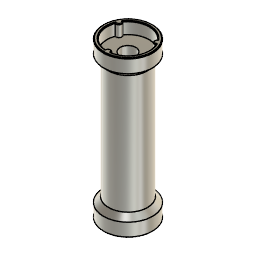
10 Spool Top Hat for Voron 2.4 - Alpha Release (Autodesk Fusion 360 archive; units mm, degrees)
design "spool roller"
Autodesk Fusion 360 part; units mm, degrees
sketch "Sketch1" plane through (0, 0, 0) normal (0, 0, 1) x (1, 0, 0)
  circle A0 centre (0, 0) radius 12.5
  circle A1 centre (0, 0) radius 14.5
  dimension "d1" = 25
  dimension "d2" = 2
  constraint coincident A0.centre A1.centre
  measures "d1" diameter of A0
extrude "Extrude1" add sketch "Sketch1" along normal blind 7
sketch "Sketch2" plane through (0, 0, 0) normal (0, 0, -1) x (1, 0, 0)
  circle A0 centre (0, 0) radius 12.5
  circle A1 centre (0, 0) radius 14.5
extrude "Extrude2" add sketch "Sketch2" along normal blind 1 contours A0 | A1
sketch "Sketch3" plane through (0, 0, -1) normal (0, 0, -1) x (1, 0, 0)
  circle A0 centre (0, 0) radius 14.5
  circle A1 centre (0, 0) radius 4.6
  dimension "d7" = 9.2
  constraint coincident A0.centre A1.centre
  measures "d7" diameter of A1
extrude "Extrude3" cut sketch "Sketch3" against normal blind 1 contours A1
sketch "Sketch4" plane through (0, 0, -1) normal (0, 0, -1) x (1, 0, 0)
  circle A0 centre (0, 0) radius 4.6
  circle A1 centre (0, 0) radius 14.5
  circle A2 centre (0, 0) radius 11.5
  dimension "d10" = 23
  constraint coincident A0.centre A1.centre
  measures "d10" diameter of A2
extrude "Extrude4" add sketch "Sketch4" along normal blind 38 contours A2
chamfer "Chamfer1" distance 3 angle 45 1 edges at (-10.7218, -4.1586, -1)
sketch "Sketch5" plane through (0, 0, 7) normal (0, 0, 1) x (-1, 0, 0)
  circle A0 centre (0, 0) radius 12.5
  circle A1 centre (0, 0) radius 14.5
  circle A2 centre (0, 0) radius 10.85
  circle A3 centre (-0.6001, 12.4856) radius 1.65
  dimension "d16" = 21.7
  constraint coincident A0.centre A1.centre
  constraint coincident A0 A3.centre
  constraint tangent A2 A3
  measures "d16" diameter of A2
extrude "Extrude5" add sketch "Sketch5" against normal blind 7 contours A0 A3 picked at (-0.5733, 11.9282)
pattern_circular "C-Pattern1" count 3 over 360 about axis through (0, 0, -39) along (0, 0, 1) of "Extrude5"
mirror "Mirror2" about plane through (0, 0, -39) normal (0, 0, -1) of bodies 1 merged
chamfer "Chamfer2" distance 0.4 angle 45 1 faces at (10.941, 7.1918, 7)
chamfer "Chamfer3" distance 0.4 angle 45 1 faces at (10.941, 7.1918, -85)

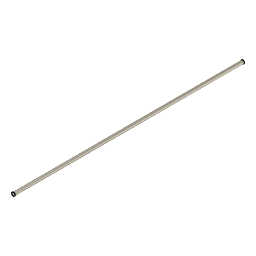
design "8x500 shaft"
Autodesk Fusion 360 part; units mm, degrees
sketch "Sketch1" plane through (0, 0, 0) normal (0, 1, 0) x (1, 0, 0)
  circle A0 centre (0, 0) radius 3.98
  dimension "d1" = 7.96
  constraint coincident A0.centre origin
  measures "d1" diameter of A0
extrude "Extrude1" add sketch "Sketch1" along normal blind 500

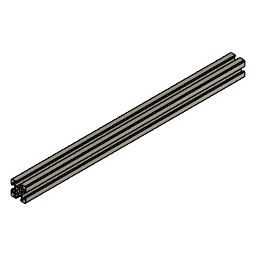
design "2020 extrusion - 300mm"
Autodesk Fusion 360 part; units mm, degrees
sketch "Sketch1" plane through (0, 0, 0) normal (0, 1, 0) x (1, 0, 0)
  arc A0 (8.9954, -10.0126) -> (9.9954, -9.0126) centre (8.9954, -9.0126) ccw
  line L0 (2.9954, 9.9874) -> (2.9954, 7.9874)
  line L1 (2.9954, -8.0126) -> (2.9954, -10.0126)
  line L2 (-8.0046, -3.0126) -> (-10.0046, -3.0126)
  line L3 (7.9954, 2.9874) -> (9.9954, 2.9874)
  line L4 (9.9954, -3.0126) -> (7.9954, -3.0126)
  line L5 (-8.0046, 2.9874) -> (-8.0046, 5.9874)
  line L6 (5.9954, -8.0126) -> (2.9954, -8.0126)
  line L7 (-4.0046, -2.952) -> (-7.0653, -6.0126)
  line L8 (-2.9439, 3.9874) -> (-6.0046, 7.048)
  line L9 (9.9954, -9.0126) -> (9.9954, -3.0126)
  line L10 (-0.5242, 3.9874) -> (-2.9439, 3.9874)
  arc A1 (8.9954, -10.0126) -> (9.9954, -9.0126) centre (8.9954, -9.0126) ccw
  line L11 (7.9954, 5.9874) -> (7.9954, 2.9874)
  line L12 (5.9954, 7.9874) -> (5.9954, 7.048)
  line L13 (3.9954, -0.5323) -> (3.6954, -0.0126)
  line L14 (-6.0046, 7.048) -> (-6.0046, 7.9874)
  line L15 (7.9954, -6.0126) -> (7.0561, -6.0126)
  circle A2 centre (-0.0046, -0.0126) radius 2.1
  line L16 (7.9954, -3.0126) -> (7.9954, -6.0126)
  line L17 (-0.5242, -4.0126) -> (-0.0046, -3.7126)
  line L18 (-6.0046, 7.048) -> (-6.0046, 7.9874)
  line L19 (-6.0046, -8.0126) -> (-6.0046, -7.0733)
  line L20 (-6.0046, 7.9874) -> (-3.0046, 7.9874)
  arc A3 (9.9954, 8.9874) -> (8.9954, 9.9874) centre (8.9954, 8.9874) ccw
  line L21 (-8.0046, -3.0126) -> (-10.0046, -3.0126)
  line L22 (3.6954, -0.0126) -> (3.9954, 0.507)
  line L23 (2.9954, 7.9874) -> (5.9954, 7.9874)
  line L24 (2.9954, -8.0126) -> (2.9954, -10.0126)
  line L25 (-4.0046, 2.9267) -> (-4.0046, 0.507)
  line L26 (7.0561, -6.0126) -> (3.9954, -2.952)
  line L27 (-8.0046, -6.0126) -> (-8.0046, -3.0126)
  line L28 (2.9347, -4.0126) -> (5.9954, -7.0733)
  line L29 (9.9954, 2.9874) -> (9.9954, 8.9874)
  line L30 (-3.0046, 7.9874) -> (-3.0046, 9.9874)
  line L31 (0.515, -4.0126) -> (2.9347, -4.0126)
  line L32 (-2.9439, -4.0126) -> (-0.5242, -4.0126)
  line L33 (-10.0046, -3.0126) -> (-10.0046, -9.0126)
  line L34 (-3.0046, 9.9874) -> (-9.0046, 9.9874)
  line L35 (3.9954, -2.952) -> (3.9954, -0.5323)
  line L36 (3.9954, 2.9267) -> (7.0561, 5.9874)
  arc A4 (-10.0046, -9.0126) -> (-9.0046, -10.0126) centre (-9.0046, -9.0126) ccw
  line L37 (7.9954, -3.0126) -> (7.9954, -6.0126)
  line L38 (5.9954, -8.0126) -> (2.9954, -8.0126)
  line L39 (9.9954, -3.0126) -> (7.9954, -3.0126)
  line L40 (2.9954, -10.0126) -> (8.9954, -10.0126)
  line L41 (-9.0046, -10.0126) -> (-3.0046, -10.0126)
  line L42 (-3.0046, -8.0126) -> (-6.0046, -8.0126)
  line L43 (2.9347, 3.9874) -> (0.515, 3.9874)
  line L44 (-4.0046, -0.5323) -> (-4.0046, -2.952)
  line L45 (9.9954, -9.0126) -> (9.9954, -3.0126)
  line L46 (-6.0046, 7.9874) -> (-3.0046, 7.9874)
  line L47 (-3.7046, -0.0126) -> (-4.0046, -0.5323)
  line L48 (-3.0046, 7.9874) -> (-3.0046, 9.9874)
  line L49 (3.9954, 0.507) -> (3.9954, 2.9267)
  line L50 (-10.0046, 8.9874) -> (-10.0046, 2.9874)
  line L51 (-0.0046, 3.6874) -> (-0.5242, 3.9874)
  line L52 (-10.0046, 2.9874) -> (-8.0046, 2.9874)
  arc A5 (-9.0046, 9.9874) -> (-10.0046, 8.9874) centre (-9.0046, 8.9874) ccw
  line L53 (-10.0046, 8.9874) -> (-10.0046, 2.9874)
  line L54 (-10.0046, 2.9874) -> (-8.0046, 2.9874)
  line L55 (3.6954, -0.0126) -> (3.9954, 0.507)
  line L56 (-3.0046, -10.0126) -> (-3.0046, -8.0126)
  line L57 (-4.0046, 0.507) -> (-3.7046, -0.0126)
  line L58 (5.9954, 7.048) -> (2.9347, 3.9874)
  line L59 (-8.0046, 2.9874) -> (-8.0046, 5.9874)
  line L60 (-4.0046, 2.9267) -> (-4.0046, 0.507)
  line L61 (7.0561, 5.9874) -> (7.9954, 5.9874)
  line L62 (-7.0653, 5.9874) -> (-4.0046, 2.9267)
  line L63 (-8.0046, 5.9874) -> (-7.0653, 5.9874)
  arc A6 (9.9954, 8.9874) -> (8.9954, 9.9874) centre (8.9954, 8.9874) ccw
  line L64 (0.515, 3.9874) -> (-0.0046, 3.6874)
  line L65 (-2.9439, 3.9874) -> (-6.0046, 7.048)
  line L66 (7.9954, 5.9874) -> (7.9954, 2.9874)
  line L67 (-6.0046, -8.0126) -> (-6.0046, -7.0733)
  line L68 (-8.0046, 5.9874) -> (-7.0653, 5.9874)
  line L69 (3.9954, -2.952) -> (3.9954, -0.5323)
  line L70 (3.9954, -0.5323) -> (3.6954, -0.0126)
  line L71 (-0.0046, 3.6874) -> (-0.5242, 3.9874)
  line L72 (-3.0046, 9.9874) -> (-9.0046, 9.9874)
  line L73 (2.9954, 9.9874) -> (2.9954, 7.9874)
  line L74 (7.0561, 5.9874) -> (7.9954, 5.9874)
  line L75 (-0.5242, 3.9874) -> (-2.9439, 3.9874)
  line L76 (2.9347, 3.9874) -> (0.515, 3.9874)
  line L77 (-6.0046, -7.0733) -> (-2.9439, -4.0126)
  line L78 (-0.0046, -3.7126) -> (0.515, -4.0126)
  line L79 (2.9954, -10.0126) -> (8.9954, -10.0126)
  line L80 (8.9954, 9.9874) -> (2.9954, 9.9874)
  line L81 (-7.0653, -6.0126) -> (-8.0046, -6.0126)
  line L82 (-4.0046, 0.507) -> (-3.7046, -0.0126)
  line L83 (5.9954, -7.0733) -> (5.9954, -8.0126)
  line L84 (3.9954, 2.9267) -> (7.0561, 5.9874)
  line L85 (5.9954, 7.048) -> (2.9347, 3.9874)
  line L86 (5.9954, 7.9874) -> (5.9954, 7.048)
  line L87 (-7.0653, 5.9874) -> (-4.0046, 2.9267)
  line L88 (-10.0046, -3.0126) -> (-10.0046, -9.0126)
  arc A7 (-9.0046, 9.9874) -> (-10.0046, 8.9874) centre (-9.0046, 8.9874) ccw
  line L89 (7.0561, -6.0126) -> (3.9954, -2.952)
  line L90 (2.9347, -4.0126) -> (5.9954, -7.0733)
  line L91 (2.9954, 7.9874) -> (5.9954, 7.9874)
  line L92 (-0.5242, -4.0126) -> (-0.0046, -3.7126)
  line L93 (9.9954, 2.9874) -> (9.9954, 8.9874)
  arc A8 (-10.0046, -9.0126) -> (-9.0046, -10.0126) centre (-9.0046, -9.0126) ccw
  line L94 (-8.0046, -6.0126) -> (-8.0046, -3.0126)
  line L95 (-0.0046, -3.7126) -> (0.515, -4.0126)
  line L96 (0.515, -4.0126) -> (2.9347, -4.0126)
  line L97 (7.9954, -6.0126) -> (7.0561, -6.0126)
  line L98 (7.9954, 2.9874) -> (9.9954, 2.9874)
  line L99 (-2.9439, -4.0126) -> (-0.5242, -4.0126)
  line L100 (3.9954, 0.507) -> (3.9954, 2.9267)
  line L101 (8.9954, 9.9874) -> (2.9954, 9.9874)
  line L102 (-7.0653, -6.0126) -> (-8.0046, -6.0126)
  line L103 (0.515, 3.9874) -> (-0.0046, 3.6874)
  line L104 (5.9954, -7.0733) -> (5.9954, -8.0126)
  line L105 (-3.7046, -0.0126) -> (-4.0046, -0.5323)
  line L106 (-3.0046, -8.0126) -> (-6.0046, -8.0126)
  line L107 (-4.0046, -2.952) -> (-7.0653, -6.0126)
  line L108 (-6.0046, -7.0733) -> (-2.9439, -4.0126)
  line L109 (-9.0046, -10.0126) -> (-3.0046, -10.0126)
  line L110 (-3.0046, -10.0126) -> (-3.0046, -8.0126)
  line L111 (-4.0046, -0.5323) -> (-4.0046, -2.952)
  dimension "d1" = 0
  measures "d1" distance of L79
extrude "Extrude1" add sketch "Sketch1" along normal blind 300

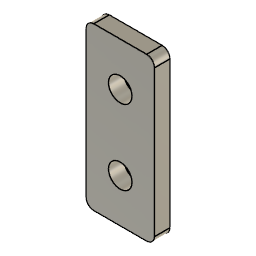
design "2020 joining plate"
Autodesk Fusion 360 part; units mm, degrees
sketch "Sketch1" plane through (0, 0, 0) normal (0, 1, 0) x (1, 0, 0)
  line L0 (8.7313, 20.6375) -> (-8.7313, 20.6375)
  line L1 (-8.7313, 20.6375) -> (-8.7313, -20.6375)
  line L2 (-8.7313, -20.6375) -> (8.7313, -20.6375)
  line L3 (8.7313, -20.6375) -> (8.7313, 20.6375)
  line L4 (8.7313, 20.6375) -> (-8.7313, -20.6375) construction
  line L5 (-8.7313, 20.6375) -> (8.7313, -20.6375) construction
  dimension "d1" = 17.4625
  dimension "d2" = 41.275
  constraint horizontal L0
  constraint perpendicular L0 L1
  constraint parallel L0 L2
  constraint parallel L1 L3
  constraint coincident L4 origin
  constraint coincident L5 origin
  measures "d1" distance of L1.end L2.end
  measures "d2" distance of L0.end L1.end
extrude "Extrude1" add sketch "Sketch1" along normal blind 3.9688
sketch "Sketch2" plane through (0, 0, 0) normal (0, -1, 0) x (1, 0, 0)
  line L0 (8.7313, -20.6375) -> (8.7313, 20.6375)
  line L1 (8.7313, 20.6375) -> (-8.7313, 20.6375)
  line L2 (-8.7313, 20.6375) -> (-8.7313, -20.6375)
  line L3 (-8.7313, -20.6375) -> (8.7313, -20.6375)
  circle A0 centre (0, 9.525) radius 3
  dimension "d5" = 6
  dimension "d6" = 9.525
  measures "d5" diameter of A0
  measures "d6" distance of origin A0.centre
extrude "Extrude2" cut sketch "Sketch2" against normal blind 15 contours A0
mirror "Mirror1" about plane through (0, 0, 0) normal (0, 0, 1) of "Extrude2"
fillet "Fillet1" radius 2 4 edges at (8.7313, 1.9844, 20.6375) (-8.7313, 1.9844, 20.6375) (-8.7313, 1.9844, -20.6375) (8.7313, 1.9844, -20.6375)
equation "d2 = 1 5/8\""
equation "d6 = 0.75 in / 2"

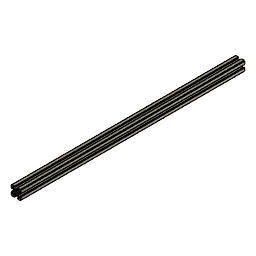
design "2020 extrusion - 470mm"
Autodesk Fusion 360 part; units mm, degrees
sketch "Sketch1" plane through (0, 0, 0) normal (0, 1, 0) x (1, 0, 0)
  arc A0 (8.9954, -10.0126) -> (9.9954, -9.0126) centre (8.9954, -9.0126) ccw
  line L0 (2.9954, 9.9874) -> (2.9954, 7.9874)
  line L1 (2.9954, -8.0126) -> (2.9954, -10.0126)
  line L2 (-8.0046, -3.0126) -> (-10.0046, -3.0126)
  line L3 (7.9954, 2.9874) -> (9.9954, 2.9874)
  line L4 (9.9954, -3.0126) -> (7.9954, -3.0126)
  line L5 (-8.0046, 2.9874) -> (-8.0046, 5.9874)
  line L6 (5.9954, -8.0126) -> (2.9954, -8.0126)
  line L7 (-4.0046, -2.952) -> (-7.0653, -6.0126)
  line L8 (-2.9439, 3.9874) -> (-6.0046, 7.048)
  line L9 (9.9954, -9.0126) -> (9.9954, -3.0126)
  line L10 (-0.5242, 3.9874) -> (-2.9439, 3.9874)
  arc A1 (8.9954, -10.0126) -> (9.9954, -9.0126) centre (8.9954, -9.0126) ccw
  line L11 (7.9954, 5.9874) -> (7.9954, 2.9874)
  line L12 (5.9954, 7.9874) -> (5.9954, 7.048)
  line L13 (3.9954, -0.5323) -> (3.6954, -0.0126)
  line L14 (-6.0046, 7.048) -> (-6.0046, 7.9874)
  line L15 (7.9954, -6.0126) -> (7.0561, -6.0126)
  circle A2 centre (-0.0046, -0.0126) radius 2.1
  line L16 (7.9954, -3.0126) -> (7.9954, -6.0126)
  line L17 (-0.5242, -4.0126) -> (-0.0046, -3.7126)
  line L18 (-6.0046, 7.048) -> (-6.0046, 7.9874)
  line L19 (-6.0046, -8.0126) -> (-6.0046, -7.0733)
  line L20 (-6.0046, 7.9874) -> (-3.0046, 7.9874)
  arc A3 (9.9954, 8.9874) -> (8.9954, 9.9874) centre (8.9954, 8.9874) ccw
  line L21 (-8.0046, -3.0126) -> (-10.0046, -3.0126)
  line L22 (3.6954, -0.0126) -> (3.9954, 0.507)
  line L23 (2.9954, 7.9874) -> (5.9954, 7.9874)
  line L24 (2.9954, -8.0126) -> (2.9954, -10.0126)
  line L25 (-4.0046, 2.9267) -> (-4.0046, 0.507)
  line L26 (7.0561, -6.0126) -> (3.9954, -2.952)
  line L27 (-8.0046, -6.0126) -> (-8.0046, -3.0126)
  line L28 (2.9347, -4.0126) -> (5.9954, -7.0733)
  line L29 (9.9954, 2.9874) -> (9.9954, 8.9874)
  line L30 (-3.0046, 7.9874) -> (-3.0046, 9.9874)
  line L31 (0.515, -4.0126) -> (2.9347, -4.0126)
  line L32 (-2.9439, -4.0126) -> (-0.5242, -4.0126)
  line L33 (-10.0046, -3.0126) -> (-10.0046, -9.0126)
  line L34 (-3.0046, 9.9874) -> (-9.0046, 9.9874)
  line L35 (3.9954, -2.952) -> (3.9954, -0.5323)
  line L36 (3.9954, 2.9267) -> (7.0561, 5.9874)
  arc A4 (-10.0046, -9.0126) -> (-9.0046, -10.0126) centre (-9.0046, -9.0126) ccw
  line L37 (7.9954, -3.0126) -> (7.9954, -6.0126)
  line L38 (5.9954, -8.0126) -> (2.9954, -8.0126)
  line L39 (9.9954, -3.0126) -> (7.9954, -3.0126)
  line L40 (2.9954, -10.0126) -> (8.9954, -10.0126)
  line L41 (-9.0046, -10.0126) -> (-3.0046, -10.0126)
  line L42 (-3.0046, -8.0126) -> (-6.0046, -8.0126)
  line L43 (2.9347, 3.9874) -> (0.515, 3.9874)
  line L44 (-4.0046, -0.5323) -> (-4.0046, -2.952)
  line L45 (9.9954, -9.0126) -> (9.9954, -3.0126)
  line L46 (-6.0046, 7.9874) -> (-3.0046, 7.9874)
  line L47 (-3.7046, -0.0126) -> (-4.0046, -0.5323)
  line L48 (-3.0046, 7.9874) -> (-3.0046, 9.9874)
  line L49 (3.9954, 0.507) -> (3.9954, 2.9267)
  line L50 (-10.0046, 8.9874) -> (-10.0046, 2.9874)
  line L51 (-0.0046, 3.6874) -> (-0.5242, 3.9874)
  line L52 (-10.0046, 2.9874) -> (-8.0046, 2.9874)
  arc A5 (-9.0046, 9.9874) -> (-10.0046, 8.9874) centre (-9.0046, 8.9874) ccw
  line L53 (-10.0046, 8.9874) -> (-10.0046, 2.9874)
  line L54 (-10.0046, 2.9874) -> (-8.0046, 2.9874)
  line L55 (3.6954, -0.0126) -> (3.9954, 0.507)
  line L56 (-3.0046, -10.0126) -> (-3.0046, -8.0126)
  line L57 (-4.0046, 0.507) -> (-3.7046, -0.0126)
  line L58 (5.9954, 7.048) -> (2.9347, 3.9874)
  line L59 (-8.0046, 2.9874) -> (-8.0046, 5.9874)
  line L60 (-4.0046, 2.9267) -> (-4.0046, 0.507)
  line L61 (7.0561, 5.9874) -> (7.9954, 5.9874)
  line L62 (-7.0653, 5.9874) -> (-4.0046, 2.9267)
  line L63 (-8.0046, 5.9874) -> (-7.0653, 5.9874)
  arc A6 (9.9954, 8.9874) -> (8.9954, 9.9874) centre (8.9954, 8.9874) ccw
  line L64 (0.515, 3.9874) -> (-0.0046, 3.6874)
  line L65 (-2.9439, 3.9874) -> (-6.0046, 7.048)
  line L66 (7.9954, 5.9874) -> (7.9954, 2.9874)
  line L67 (-6.0046, -8.0126) -> (-6.0046, -7.0733)
  line L68 (-8.0046, 5.9874) -> (-7.0653, 5.9874)
  line L69 (3.9954, -2.952) -> (3.9954, -0.5323)
  line L70 (3.9954, -0.5323) -> (3.6954, -0.0126)
  line L71 (-0.0046, 3.6874) -> (-0.5242, 3.9874)
  line L72 (-3.0046, 9.9874) -> (-9.0046, 9.9874)
  line L73 (2.9954, 9.9874) -> (2.9954, 7.9874)
  line L74 (7.0561, 5.9874) -> (7.9954, 5.9874)
  line L75 (-0.5242, 3.9874) -> (-2.9439, 3.9874)
  line L76 (2.9347, 3.9874) -> (0.515, 3.9874)
  line L77 (-6.0046, -7.0733) -> (-2.9439, -4.0126)
  line L78 (-0.0046, -3.7126) -> (0.515, -4.0126)
  line L79 (2.9954, -10.0126) -> (8.9954, -10.0126)
  line L80 (8.9954, 9.9874) -> (2.9954, 9.9874)
  line L81 (-7.0653, -6.0126) -> (-8.0046, -6.0126)
  line L82 (-4.0046, 0.507) -> (-3.7046, -0.0126)
  line L83 (5.9954, -7.0733) -> (5.9954, -8.0126)
  line L84 (3.9954, 2.9267) -> (7.0561, 5.9874)
  line L85 (5.9954, 7.048) -> (2.9347, 3.9874)
  line L86 (5.9954, 7.9874) -> (5.9954, 7.048)
  line L87 (-7.0653, 5.9874) -> (-4.0046, 2.9267)
  line L88 (-10.0046, -3.0126) -> (-10.0046, -9.0126)
  arc A7 (-9.0046, 9.9874) -> (-10.0046, 8.9874) centre (-9.0046, 8.9874) ccw
  line L89 (7.0561, -6.0126) -> (3.9954, -2.952)
  line L90 (2.9347, -4.0126) -> (5.9954, -7.0733)
  line L91 (2.9954, 7.9874) -> (5.9954, 7.9874)
  line L92 (-0.5242, -4.0126) -> (-0.0046, -3.7126)
  line L93 (9.9954, 2.9874) -> (9.9954, 8.9874)
  arc A8 (-10.0046, -9.0126) -> (-9.0046, -10.0126) centre (-9.0046, -9.0126) ccw
  line L94 (-8.0046, -6.0126) -> (-8.0046, -3.0126)
  line L95 (-0.0046, -3.7126) -> (0.515, -4.0126)
  line L96 (0.515, -4.0126) -> (2.9347, -4.0126)
  line L97 (7.9954, -6.0126) -> (7.0561, -6.0126)
  line L98 (7.9954, 2.9874) -> (9.9954, 2.9874)
  line L99 (-2.9439, -4.0126) -> (-0.5242, -4.0126)
  line L100 (3.9954, 0.507) -> (3.9954, 2.9267)
  line L101 (8.9954, 9.9874) -> (2.9954, 9.9874)
  line L102 (-7.0653, -6.0126) -> (-8.0046, -6.0126)
  line L103 (0.515, 3.9874) -> (-0.0046, 3.6874)
  line L104 (5.9954, -7.0733) -> (5.9954, -8.0126)
  line L105 (-3.7046, -0.0126) -> (-4.0046, -0.5323)
  line L106 (-3.0046, -8.0126) -> (-6.0046, -8.0126)
  line L107 (-4.0046, -2.952) -> (-7.0653, -6.0126)
  line L108 (-6.0046, -7.0733) -> (-2.9439, -4.0126)
  line L109 (-9.0046, -10.0126) -> (-3.0046, -10.0126)
  line L110 (-3.0046, -10.0126) -> (-3.0046, -8.0126)
  line L111 (-4.0046, -0.5323) -> (-4.0046, -2.952)
  dimension "d1" = 0
  measures "d1" distance of L79
extrude "Extrude1" add sketch "Sketch1" along normal blind 470
